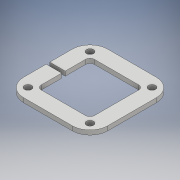
# Autodesk Inventor part: NewFront_E
Saved by Autodesk Inventor 2017 (Build 210142000, 142)
## iProperties
Created: 2019-12-01
Part Number: NewFront_E
Material: Generic
Document SubType Name: Modeling
Designer: DDeGo
Density: 1 g/cm^3
Appearance: Default
Author: DDeGo
Autodesk Inventor part; units mm, degrees
ref_plane "YZ Plane" through (0, 0, 0) normal (1, 0, 0) x (0, 1, 0)
ref_plane "XZ Plane" through (0, 0, 0) normal (0, 1, 0) x (-1, 0, 0)
ref_plane "XY Plane" through (0, 0, 0) normal (0, 0, 1) x (1, 0, 0)
sketch "Sketch1" plane through (0, 0, 0) normal (0, 0, 1) x (1, 0, 0)
  line L0 (-27.45, -52.45) -> (27.45, -52.45) construction
  line L1 (52.45, -27.45) -> (52.45, 27.45) construction
  line L2 (27.45, 52.45) -> (-27.45, 52.45) construction
  line L3 (-52.45, 27.45) -> (-52.45, -27.45) construction
  line L4 (-52.45, -52.45) -> (52.45, 52.45) construction
  line L5 (52.45, -52.45) -> (-52.45, 52.45) construction
  arc A0 (-27.45, 52.45) -> (-52.45, 27.45) centre (-27.45, 27.45) ccw construction
  arc A1 (-52.45, -27.45) -> (-27.45, -52.45) centre (-27.45, -27.45) ccw construction
  arc A2 (27.45, -52.45) -> (52.45, -27.45) centre (27.45, -27.45) ccw construction
  arc A3 (52.45, 27.45) -> (27.45, 52.45) centre (27.45, 27.45) ccw construction
  line L6 (47.45, 27.45) -> (47.45, -27.45)
  arc A4 (27.45, -47.45) -> (47.45, -27.45) centre (27.45, -27.45) ccw
  line L7 (27.45, -47.45) -> (-27.45, -47.45)
  arc A5 (-47.45, -27.45) -> (-27.45, -47.45) centre (-27.45, -27.45) ccw
  line L8 (-47.45, -27.45) -> (-47.45, 27.45)
  arc A6 (-27.45, 47.45) -> (-47.45, 27.45) centre (-27.45, 27.45) ccw
  line L9 (-27.45, 47.45) -> (27.45, 47.45)
  arc A7 (47.45, 27.45) -> (27.45, 47.45) centre (27.45, 27.45) ccw
  line L10 (-35, 35) -> (35, 35) construction
  line L11 (35, 35) -> (35, -35) construction
  line L12 (35, -35) -> (-35, -35) construction
  line L13 (-35, -35) -> (-35, 35) construction
  line L14 (-35, 35) -> (35, -35) construction
  line L15 (35, 35) -> (-35, -35) construction
  circle A8 centre (35, 35) radius 4
  circle A9 centre (35, -35) radius 4
  circle A10 centre (-35, -35) radius 4
  circle A11 centre (-35, 35) radius 4
  point P0 (0, 0)
  dimension "d0" = 104.9
  dimension "d1" = 104.9
  dimension "d2" = 25
  dimension "d6" = 5
  dimension "d12" = 70
  dimension "d13" = 8
  constraints: 32 end point, 16 point on circle, 12 centre point, 9 point on line, 8 tangent, 6 equal radius, 6 parallel, 4 coincident, 4 midpoint, 3 perpendicular, 2 horizontal, 7 other
  measures "d0" distance between parallel lines of L3 L1
  measures "d1" distance between parallel lines of L2 L0
  measures "d2" radius of A0
  measures "d6" distance between parallel lines of L1 L6
  measures "d12" distance of L10.end L11.end
  measures "d13" diameter of A8
extrude "Extrusion1" add sketch "Sketch1" along normal blind 5
sketch "Sketch2" plane through (0, 0, 5) normal (0, 0, 1) x (1, 0, 0)
  line L0 (-30, 30) -> (30, 30)
  line L1 (30, 30) -> (30, -30)
  line L2 (30, -30) -> (-30, -30)
  line L3 (-30, 30) -> (30, -30) construction
  line L4 (30, 30) -> (-30, -30) construction
  line L5 (-64.9, 2) -> (-30, 2)
  line L6 (-30, -2) -> (-64.9, -2)
  line L7 (-64.9, -2) -> (-64.9, 2)
  line L8 (-47.45, 27.45) -> (-47.45, -27.45) projected
  line L9 (-64.9, 2) -> (-30, -2) construction
  line L10 (-30, 2) -> (-64.9, -2) construction
  line L11 (-30, -30) -> (-30, -2)
  line L12 (-30, 2) -> (-30, 30)
  point P0 (0, 0)
  point P1 (-47.45, 0)
  dimension "d7" = 4
  dimension "d8" = 60
  dimension "d9" = 60
  constraints: 24 end point, 5 midpoint, 4 parallel, 2 horizontal, 1 collinear, 1 perpendicular, 1 vertical
  measures "d7" distance of L6.end L5.start
  measures "d8" distance between parallel lines of L0 L2
  measures "d9" distance of L1.end L2.end
extrude "Extrusion2" cut sketch "Sketch2" against normal blind 10
fillet "Fillet1" radius 5 4 edges at (30, 30, 2.5) (-30, 30, 2.5) (30, -30, 2.5) (-30, -30, 2.5)
equation "\"d1\" = d0"
equation "\"d8\" = d9"
body "Solid1"
